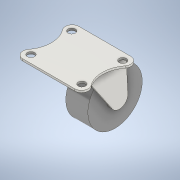
# Autodesk Inventor part: Castor_Wheel
Saved by Autodesk Inventor 2021 (Build 250183000, 183)
## iProperties
Created: 2021-06-13
Part Number: Castor_Wheel
Material: Stahl, unlegiert
Document SubType Name: Modeling
Designer: User
Mass: 113.562 g
Surface Area: 73.2002 cm^2
Volume: 14.4665 cm^3
Density: 7.85 g/cm^3
Appearance: Stahl
Author: User
Autodesk Inventor part; units mm, degrees
ref_plane "YZ Plane" through (0, 0, 0) normal (1, 0, 0) x (0, 1, 0)
ref_plane "XZ Plane" through (0, 0, 0) normal (0, 1, 0) x (-1, 0, 0)
ref_plane "XY Plane" through (0, 0, 0) normal (0, 0, 1) x (1, 0, 0)
sketch "Skizze1" plane through (0, 0, 0) normal (0, 1, 0) x (-1, 0, 0)
  line L0 (15.25, -16.5) -> (-15.25, -16.5)
  line L1 (15.25, 16.5) -> (-15.25, 16.5)
  arc A0 (-18.421, -10.0619) -> (-18.421, 10.0619) centre (-31.5074, 0) ccw
  arc A1 (18.421, 10.0619) -> (18.421, -10.0619) centre (31.5074, 0) ccw
  arc A2 (15.25, -16.5) -> (18.421, -10.0619) centre (15.25, -12.5) ccw
  arc A3 (18.421, 10.0619) -> (15.25, 16.5) centre (15.25, 12.5) ccw
  arc A4 (-15.25, 16.5) -> (-18.421, 10.0619) centre (-15.25, 12.5) ccw
  arc A5 (-18.421, -10.0619) -> (-15.25, -16.5) centre (-15.25, -12.5) ccw
  circle A6 centre (15, -12) radius 2.15
  circle A7 centre (-15, -12) radius 2.15
  circle A8 centre (-15, 12) radius 2.15
  circle A9 centre (15, 12) radius 2.15
  line L2 (15, 12) -> (15, -12) construction
  line L3 (15, -12) -> (-15, -12) construction
  line L4 (-15, -12) -> (-15, 12) construction
  line L5 (-15, 12) -> (15, 12) construction
  line L6 (0, -24.4811) -> (0, 24.4811) projected
  line L7 (44.8, 0) -> (-44.8, 0) projected
  line L8 (15, 0) -> (-15, 0) construction
  point P0 (0, 0)
  point P1 (32, -16.5)
  point P2 (-32, -16.5)
  point P3 (32, 16.5)
  point P4 (-32, 16.5)
  dimension "d0" = 4
  dimension "d1" = 30
  dimension "d2" = 24
  dimension "d3" = 33
  dimension "d4" = 4.3
  dimension "d5" = 38.5
  constraints: 18 point on circle, 14 end point, 10 centre point, 8 tangent, 6 equal radius, 6 point on line, 2 horizontal, 2 perpendicular, 1 parallel, 1 vertical, 1 vertical alignment, 4 other
  measures "d0" radius of A2
  measures "d1" distance of L2.end L3.end
  measures "d2" distance of L3.end L4.end
  measures "d3" distance between parallel lines of L0 L1
  measures "d4" diameter of A6
extrude "Extrusion1" add sketch "Skizze1" along normal blind 1.2
sketch "Skizze2" plane through (0, 0, 0) normal (1, 0, 0) x (0, 1, 0)
  line L0 (0, 10.0619) -> (0, -10.0619) projected
  line L1 (0, 12) -> (-3, 12)
  line L2 (-3, 12) -> (-3, -12)
  line L3 (-3, -12) -> (0, -12)
  line L4 (-1.683, 0) -> (1.6805, 0) projected
  circle A0 centre (-23.6, -16) radius 16
  line L5 (1.2, 10.0619) -> (1.2, -10.0619) projected
  line L6 (0, -16.5) -> (1.2, -16.5) projected
  circle A1 centre (-23.6, -16) radius 5
  line L7 (-3, -12) -> (-3, -20)
  line L8 (-3, -20) -> (-23.3561, -20.994)
  line L9 (-3, 4) -> (-26.405, -11.8609)
  line L10 (0, 0) -> (-3, 0)
  line L11 (0, 10.0619) -> (0, -10.0619) projected
  line L12 (0, 0) -> (0, -12)
  dimension "d8" = 3
  dimension "d9" = 32
  dimension "d10" = 40.8
  dimension "d12" = 0
  dimension "d13" = 10
  dimension "d14" = 8
  dimension "d16" = 8
  dimension "d18" = 24
  constraints: 16 end point, 5 point on line, 3 perpendicular, 2 centre point, 2 point on circle, 2 tangent, 1 coincident, 1 horizontal, 1 midpoint, 1 vertical, 1 other
  measures "d8" distance between parallel lines of L0 L2
  measures "d9" diameter of A0
  measures "d12" distance edge to line of A0 L4
  measures "d13" diameter of A1
  measures "d14" distance of L2.end L7.end
  measures "d16" distance from line of L1 L9.start
  measures "d18" diameter of L3 L10
revolve "Umdrehung1" add sketch "Skizze2" angle 360 about axis through (0, 0, 0) along (0, -1, 0) contours L0 L12 L3 L2 L10 L4
extrude "Extrusion2" add sketch "Skizze2" along normal mid plane 13 contours L9 A1 L8 A0 | A0 L8 A1 L9
extrude "Extrusion3" add sketch "Skizze2" along normal mid plane 18 contours A1
sketch "Skizze3" plane through (-9, -23.6, -16) normal (-1, 0, 0) x (0, 0, 1)
  line L0 (-4, 20.6) -> (-4.994, 0.2439) projected
  line L1 (4, 20.6) -> (-4, 20.6) projected
  line L2 (20, 20.6) -> (4.1391, -2.805) projected
  circle A0 centre (0, 0) radius 5 projected
  line L3 (-4, 20.6) -> (20, 20.6)
  line L4 (4, 20.6) -> (28, 20.6) projected
  line L5 (20, 20.6) -> (4.1391, -2.805)
  circle A1 centre (0, 0) radius 5 projected
  arc A2 (4.1391, -2.805) -> (-4.994, 0.2439) centre (0, 0) ccw
  line L6 (-4.994, 0.2439) -> (-4, 20.6)
  point P0 (16, 23.6)
  constraints: 6 end point, 3 tangent, 2 collinear, 2 point on circle, 1 centre point
extrude "Extrusion4" add sketch "Skizze3" against normal blind 1.2 contours L1 L3 L2 A0 L0
mirror "Spiegeln1" about plane through (0, 0, 0) normal (1, 0, 0) of "Extrusion4"
sketch "Skizze4" plane through (7.8, -3, -9.1192) normal (-1, 0, 0) x (0, 0, 1)
  line L0 (-10.8808, 0) -> (-11.8748, -20.3561) projected
  line L1 (-10.9394, -1.2) -> (0, -1.2)
  line L2 (0, 0) -> (1.182, 0) projected
  line L3 (0, -1.2) -> (0, 0)
  line L4 (1.182, 0) -> (-10.8808, 0) projected
  point P0 (9.1192, 3)
  dimension "d27" = 1.2
  constraints: 4 end point, 1 horizontal, 1 perpendicular, 1 point on line
  measures "d27" distance between parallel lines of L4 L1
extrude "Extrusion5" add sketch "Skizze4" along normal up to surface (15.6 mm away)
